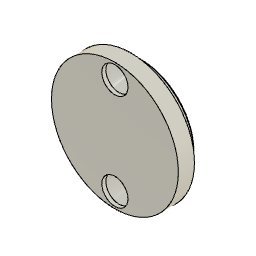
cover (Autodesk Fusion 360 design; units mm, degrees)
Autodesk Fusion 360 part; units mm, degrees
note: some values were not read from the file. Chosen so that the rebuilt part matches the saved one: which face or edge a step refers to. Set by a fixed rule: which sketch regions a step uses.
sketch "Skizze1" plane through (0, -3, 0) normal (0, -1, 0) x (1, 0, 0)
  circle A0 centre (0, 0) radius 14
  circle A1 centre (0, 0) radius 15.75
  circle A2 centre (0, 12) radius 2.35
  line L0 (0, 0) -> (-10, 0)
  circle A3 centre (0, -12) radius 2.35
  arc A4 (-5.4181, 12.9091) -> (5.4181, 12.9091) centre (0, 14.5348) ccw
  circle A5 centre (0, -12) radius 2.35
  arc A6 (5.4181, -12.9091) -> (-5.4181, -12.9091) centre (0, -14.5348) ccw
  line L1 (-11.3472, -8.2) -> (11.3472, -8.2)
  circle A7 centre (0, 12) radius 1.6
  circle A8 centre (0, -12) radius 1.6
  arc A9 (-5.6097, 12.8516) -> (5.6097, 12.8516) centre (0, 14.5348) ccw
  circle A10 centre (0, 0) radius 13.65
  line L2 (-11.3472, -8) -> (11.3472, -8)
  circle A11 centre (0, 0) radius 15.25
  circle A12 centre (0, 0) radius 14
  dimension "d1" = 4.7
  dimension "d2" = 12
  dimension "d3" = 14.5348
  dimension "d4" = 8.2
  dimension "d5" = 3.2
  dimension "d6" = 0.2
  dimension "d7" = -0.35
  dimension "d8" = -0.2
  dimension "d9" = 30.5
  dimension "d10" = -1.25
  constraint vertical A0.centre A2.centre
  constraint symmetric A2 L0 A3
  constraint coincident A0 A4.end
  constraint coincident A0 A4.start
  constraint symmetric A2 L0 A5
  constraint symmetric L0 A4.start A6.end
  constraint symmetric L0 A4.end A6.start
  constraint symmetric L0 A4 A6
  constraint coincident A0 L1.start
  constraint coincident A0 L1.end
  constraint horizontal L1
  constraint concentric A2 A7
  constraint symmetric L0 A7 A8
  constraint coincident A0.centre A1.centre
  measures "d1" diameter of A2
  measures "d2" distance of A0.centre A2.centre
  measures "d3" distance of A0.centre A4.centre
  measures "d4" distance of L1 A0.centre
  measures "d5" diameter of A7
  measures "d9" diameter of A11
sketch "Skizze2" plane through (0, -4.8, 11.2915) normal (0, -1, 0) x (1, 0, 0)
  circle A0 centre (0, 0.7) radius 1.5
  line L0 (2.5, -11.2915) -> (20, -11.2915)
  circle A1 centre (0, -23.2829) radius 1.5
  dimension "d11" = 3
  constraint symmetric A0 L0 A1
  measures "d11" diameter of A0
sketch "Skizze3" plane through (0, -6, 0) normal (0, -1, 0) x (1, 0, 0)
  circle A0 centre (0, -12) radius 1.6
  circle A1 centre (0, 12) radius 1.6
  circle A2 centre (0, 0) radius 15.75
  circle A3 centre (0, -12) radius 3.25
  line L0 (2.5, 0) -> (20, 0)
  circle A4 centre (0, 12) radius 3.25
  dimension "d12" = 6.5
  constraint concentric A0 A3
  constraint symmetric A3 L0 A4
  measures "d12" diameter of A3
extrude "Extrusion1" add sketch "Skizze1" along normal blind 3 contours A0 A6 L1 A10 A12 | A0 L1 A9 A10 A12 | A0 A3 A5 A6 A10 A12 | A0 A4 A9 A10 A12 | L1 A10 L2 | A6 L1 A10 | A0 A3 A5 A10 A12 | A0 A3 A5 A12 | A3 A5 A6 A10 | A0 A2 A4 A10 A12 | A4 A9 A10 | A9 A10 L2 | A0 L1 A9 A10 A12 | A0 A6 L1 A10 A12 | A0 A3 A5 A6 A10 A12 | A3 A5 A10 | A0 A2 A12 | A0 A2 A10 A12 | A2 A4 A10 | A0 A4 A9 A10 A12 | A0 A2 A4 A10 A12 | A2 A10 | A1 | A11
extrude "Extrusion3" [suppressed]
fillet "Abrundung2" [suppressed]
loft "Erhebung3" [suppressed]
mirror "Spiegeln1" [suppressed]
sketch "Skizze4" plane through (0, -3, 0) normal (0, 1, 0) x (-1, 0, 0)
  circle A0 centre (0, 12) radius 1.6
  circle A1 centre (0, -12) radius 1.6
  circle A2 centre (0, 0) radius 15.75
  circle A3 centre (0, 0) radius 13.85
  circle A4 centre (0, 0) radius 14.85
  dimension "d13" = 27.7
  dimension "d14" = 1
  constraint concentric A2 A3
  measures "d13" diameter of A3
extrude "Extrusion5" add sketch "Skizze4" along normal blind 2.5 contours A3
chamfer "Fase2" distance 0.75 angle 45 1 edges at (12.9127, -0.5, -5.0084)
ref_plane "Arbeitsebene1" through (0, -3.5, 11.2915) normal (0, -1, 0) x (1, 0, 0)
sketch "Skizze5" plane through (0, -3.5, 11.2915) normal (0, -1, 0) x (1, 0, 0)
  circle A0 centre (0, 0.7) radius 1.6
  line L0 (0, -11.2915) -> (-10, -11.2915)
  circle A1 centre (0, -23.2829) radius 1.6
  dimension "d19" = 3.2
  constraint symmetric A0 L0 A1
  measures "d19" diameter of A0
loft "Erhebung4" cut profiles "Skizze5", "Skizze3" section 1 contours A0 section 2 contours A4
mirror "Spiegeln2" about plane through (0, 0, 0) normal (0, 0, 1) of 1 faces at (-2.6912, -5.1671, 12.2181)
extrude "Extrusion6" cut sketch "Skizze1" against normal blind 2.5 contours A0 A6 L1 A10 A12 | A0 L1 A9 A10 A12 | A0 A3 A5 A6 A10 A12 | A0 A4 A9 A10 A12 | A0 A3 A5 A10 A12 | A0 A2 A4 A10 A12 | A0 L1 A9 A10 A12 | A0 A6 L1 A10 A12 | A0 A3 A5 A6 A10 A12 | A0 A2 A10 A12 | A0 A4 A9 A10 A12 | A0 A2 A4 A10 A12
extrude "Extrusion7" add 1 faces at (-6.0416, -6, 0) along direction (0, -1, 0) blind 1
